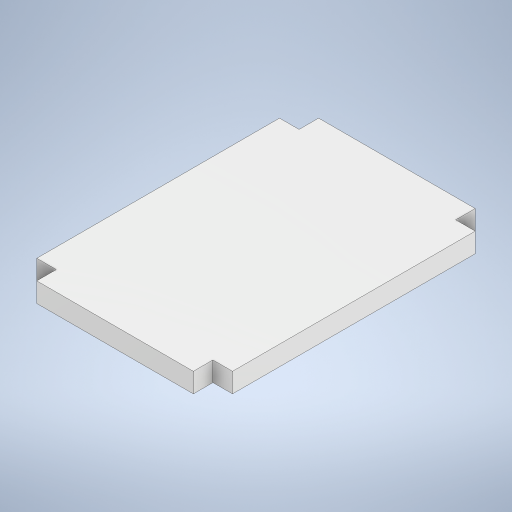
# Autodesk Inventor part: Base Plate Wall
Saved by Autodesk Inventor 2023 (Build 270158000, 158)
## iProperties
Created: 2023-02-13
Part Number: Base Plate Wall
Material: LCP Plastic
Document SubType Name: Modeling
Designer: cheng
Density: 1.626 g/cm^3
Appearance: Smooth - White
Author: cheng
Autodesk Inventor part; units mm, degrees
ref_plane "YZ Plane" through (0, 0, 0) normal (1, 0, 0) x (0, 1, 0)
ref_plane "XZ Plane" through (0, 0, 0) normal (0, 1, 0) x (-1, 0, 0)
ref_plane "XY Plane" through (0, 0, 0) normal (0, 0, 1) x (1, 0, 0)
sketch "Sketch1" plane through (0, 0, 0) normal (0, 1, 0) x (-1, 0, 0)
  line L0 (25, -31) -> (-25, -31)
  line L1 (-25, -31) -> (-25, 31)
  line L2 (-25, 31) -> (25, 31)
  line L3 (25, 31) -> (25, -31)
  line L4 (25, -31) -> (-25, 31) construction
  line L5 (-25, -31) -> (25, 31) construction
  line L6 (-20, -36) -> (20, -36)
  line L7 (20, -36) -> (20, -31)
  line L8 (20, -31) -> (-20, -31)
  line L9 (-20, -31) -> (-20, -36)
  line L10 (-20, -36) -> (20, -31) construction
  line L11 (20, -36) -> (-20, -31) construction
  line L12 (-20, 31) -> (20, 31)
  line L13 (20, 31) -> (20, 36)
  line L14 (20, 36) -> (-20, 36)
  line L15 (-20, 36) -> (-20, 31)
  line L16 (-20, 31) -> (20, 36) construction
  line L17 (20, 31) -> (-20, 36) construction
  line L18 (0, 0) -> (0, -31) construction
  line L19 (0, -33.5) -> (0, -36) construction
  line L20 (0, 33.5) -> (0, 31) construction
  point P0 (-20, 31)
  point P1 (-20, -31)
  point P2 (20, -31)
  point P3 (20, 31)
  dimension "d0" = 5
  dimension "d1" = 5
  dimension "d2" = 40
  dimension "d3" = 40
  dimension "d4" = 62
  dimension "d5" = 50
  constraints: 42 end point, 9 midpoint, 6 parallel, 4 collinear, 4 perpendicular, 3 horizontal
  measures "d0" distance of L14.end L12.start
  measures "d1" distance of L8.end L6.start
  measures "d2" distance of L13.end L14.end
  measures "d3" distance of L6.start L6.end
  measures "d4" distance of L0.end L1.end
  measures "d5" distance between parallel lines of L1 L3
extrude "Extrusion1" add sketch "Sketch1" along normal blind 5
body "Solid1"
